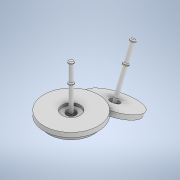
# Autodesk Inventor part: DLFinal
Saved by Autodesk Inventor 2020 (Build 240168000, 168)
## iProperties
Created: 2019-06-16
Part Number: DLFinal
Material: Generic
Document SubType Name: Modeling
Designer: Vivek Muskan
Density: 1 g/cm^3
Appearance: Default
Author: Vivek Muskan
Autodesk Inventor part; units mm, degrees
sketch "Sketch1" plane through (0, 0, 0) normal (0, 1, 0) x (-1, 0, 0)
  line L0 (0, 0) -> (0, 51)
  circle A0 centre (0, 51) radius 51
  dimension "d0" = 51
  dimension "d1" = 102
  constraints: 2 end point, 1 centre point, 1 coincident, 1 vertical
  measures "d0" distance of L0.start L0.end
  measures "d1" diameter of A0
ref_plane "Work Plane1" through (0, -10, 0) normal (0, 1, 0) x (-1, 0, 0)
sketch "Sketch2" plane through (0, -10, 0) normal (0, 1, 0) x (-1, 0, 0)
  line L0 (0, 0) -> (0, 51)
  circle A0 centre (0, 51) radius 49
  dimension "d3" = 51
  dimension "d4" = 98
  constraints: 2 end point, 1 centre point, 1 coincident, 1 vertical
  measures "d3" distance of L0.start L0.end
  measures "d4" diameter of A0
loft "Loft1" add profiles "Sketch1", "Sketch2"
sketch "Sketch3" plane through (0, 0, 51) normal (0, 1, 0) x (1, 0, 0)
  circle A0 centre (0, 0) radius 10
  circle A1 centre (0, 0) radius 3.5
  circle A2 centre (0, 0) radius 5
  line L0 (0, 0) -> (51, 0)
  circle A3 centre (0, 0) radius 51 projected
  point P0 (0, 51)
  point P1 (0, 51)
  dimension "d9" = 20
  dimension "d10" = 7
  dimension "d11" = 10
  constraints: 4 coincident, 3 centre point, 2 end point, 1 horizontal, 1 point on circle
  measures "d9" diameter of A0
  measures "d10" diameter of A1
  measures "d11" diameter of A2
extrude "Extrusion1" add sketch "Sketch3" against normal blind 20 contours A1 | A2
extrude "Extrusion2" cut sketch "Sketch3" against normal blind 20 contours A1
extrude "Extrusion3" cut sketch "Sketch3" against normal blind 5 contours A0 | A2
sketch "Sketch4" plane through (0, 0, 0) normal (1, 0, 0) x (0, 1, 0)
  line L0 (-10, 2) -> (-10, 100) projected
  line L1 (-10, 51) -> (-15, 51)
  circle A0 centre (-15, 51) radius 1.5
  point P0 (0, 0)
  dimension "d18" = 5
  dimension "d19" = 3
  constraints: 2 end point, 1 centre point, 1 coincident, 1 horizontal, 1 midpoint
  measures "d18" distance of L1.start L1.end
  measures "d19" diameter of A0
extrude "Extrusion4" cut sketch "Sketch4" against normal mid plane 12
ref_plane "BisectorPlane" through (0, 0.1961, 0.9806) normal (0, -0.1961161, -0.9805807) x (1, 0, 0)
ref_plane "Work Plane2" through (0, 0, 0) normal (0, -0.1961161, -0.9805807) x (1, 0, 0)
extrude "Extrusion5" add sketch "Sketch3" along normal blind 7 and the other way blind 20 contours A1
sketch "Sketch5" plane through (0, 7, 51) normal (0, 1, 0) x (1, 0, 0)
  circle A0 centre (0, 0) radius 4
  point P0 (0, 51)
  dimension "d27" = 8
  constraints: 1 centre point
  measures "d27" diameter of A0
extrude "Extrusion6" add sketch "Sketch5" along normal blind 100
ref_plane "Work Plane4" through (0, 62, 51) normal (0, -1, 0) x (1, 0, 0)
sketch "Sketch6" plane through (0, 62, 51) normal (0, -1, 0) x (1, 0, 0)
  circle A0 centre (0, 0) radius 10 projected
  circle A1 centre (0, 0) radius 4
  circle A2 centre (0, 0) radius 3.5 projected
  circle A3 centre (0, 0) radius 6
  point P0 (0, -51)
  dimension "d31" = 8
  dimension "d32" = 12
  constraints: 2 centre point, 2 coincident
  measures "d31" diameter of A1
  measures "d32" diameter of A3
extrude "Extrusion7" add sketch "Sketch6" against normal blind 5 contours A3
fillet "Fillet1" radius 2 2 edges at (-6, 67, 51) (-6, 62, 51)
sketch "Sketch7" plane through (0, 107, 51) normal (0, 1, 0) x (1, 0, 0)
  circle A0 centre (0, 0) radius 5 projected
  circle A1 centre (0, 0) radius 4
  circle A2 centre (0, 0) radius 6
  point P0 (0, 51)
  dimension "d36" = 8
  dimension "d37" = 12
  constraints: 2 centre point, 2 coincident
  measures "d36" diameter of A1
  measures "d37" diameter of A2
extrude "Extrusion8" add sketch "Sketch7" against normal blind 5 contours A0 | A2
fillet "Fillet2" radius 2 2 edges at (-6, 107, 51) (-6, 102, 51)
mirror "Mirror3" about plane through (0, 0.1961, 0.9806) normal (0, -0.1961161, -0.9805807) of "Loft1", "Extrusion5", "Extrusion3", "Extrusion4", "Extrusion1", "Extrusion8", "Fillet1", "Extrusion6", "Fillet2", "Extrusion7"
ref_plane "Work Plane6" through (0, 2, 51) normal (0, 1, 0) x (1, 0, 0)
sketch "Sketch8" plane through (0, 2, 51) normal (0, 1, 0) x (1, 0, 0)
  circle A0 centre (0, 0) radius 4 projected
  circle A1 centre (0, 0) radius 60
  circle A2 centre (0, 0) radius 20
  circle A3 centre (0, 0) radius 10
  point P0 (0, 51)
  dimension "d42" = 120
  dimension "d43" = 40
  dimension "d44" = 20
  constraints: 3 centre point, 3 coincident
  measures "d42" diameter of A1
  measures "d43" diameter of A2
  measures "d44" diameter of A3
extrude "Extrusion9" add sketch "Sketch8" along normal blind 10 contours A1
extrude "Extrusion10" add sketch "Sketch8" along normal blind 5 contours A2
ref_plane "Work Plane5" through (0, 38.0076, -68.9619) normal (0, 0.9230769, -0.3846154) x (1, 0, 0)
body "Solid1"
